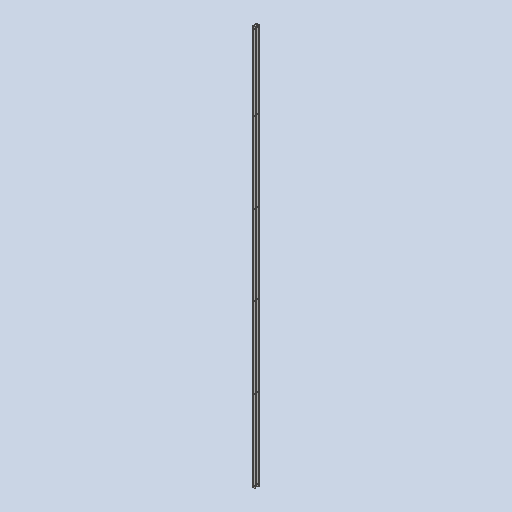
# Autodesk Inventor part: prowadnica_profil_c
Saved by Autodesk Inventor 2025.2 (Build 292293000, 293)
## iProperties
Created: 2025-03-20
Part Number: prowadnica_profil_c
Material: Ogólny
Document SubType Name: Modeling
Designer: tadek
Density: 1 g/cm^3
Appearance: Domyślna
Author: tadek
Autodesk Inventor part; units mm, degrees
ref_plane "YZ Plane" through (0, 0, 0) normal (1, 0, 0) x (0, 1, 0)
ref_plane "XZ Plane" through (0, 0, 0) normal (0, 1, 0) x (-1, 0, 0)
ref_plane "XY Plane" through (0, 0, 0) normal (0, 0, 1) x (1, 0, 0)
sketch "Szkic1" plane through (0, 0, 0) normal (0, 1, 0) x (-1, 0, 0)
  line L0 (0, 0) -> (0, -5)
  line L1 (0, -5) -> (-6, -5)
  line L2 (-6, -5) -> (-6, -3.5)
  line L3 (-6, -3.5) -> (-1.5, -3.5)
  line L4 (-1.5, -3.5) -> (-1.5, 0)
  line L5 (0, 0) -> (-1.5, 0)
  line L6 (0, 0) -> (0, 5)
  line L7 (0, 5) -> (-6, 5)
  line L8 (-6, 5) -> (-6, 3.5)
  line L9 (-6, 3.5) -> (-1.5, 3.5)
  line L10 (-1.5, 3.5) -> (-1.5, 0)
  dimension "d0" = 5
  dimension "d1" = 6
  dimension "d3" = 1.5
  dimension "d41" = 1.5
  constraints: 22 end point, 4 symmetric about line, 3 perpendicular, 2 vertical, 1 horizontal
  measures "d0" distance of L0.start L0.end
  measures "d1" distance of L0.end L1.end
  measures "d3" distance of L1.end L2.end
  measures "d41" distance between parallel lines of L0 L4
extrude "Wyciągnięcie proste1" add sketch "Szkic1" along normal blind 1000
sketch "Szkic2" plane through (1.5, 0, -3.5) normal (1, 0, 0) x (0, 0, -1)
  line L0 (-3.5, 0) -> (-3.5, 1000)
  line L1 (-7, 0) -> (-7, 1000) projected
  line L2 (-3.5, 1000) -> (-3.5, 995)
  line L3 (-3.5, 995) -> (-3.5, 795)
  line L4 (-3.5, 795) -> (-3.5, 795)
  line L5 (-3.5, 795) -> (-3.5, 695)
  line L6 (-3.5, 695) -> (-3.5, 595)
  line L7 (-3.5, 595) -> (-3.5, 495)
  line L8 (-7, 0) -> (0, 0) projected
  line L9 (-3.5, 595) -> (-3.5, 395)
  line L10 (-3.5, 395) -> (-3.5, 195)
  line L11 (-3.5, 195) -> (-3.5, 0)
  line L12 (-3.5, 0) -> (-3.5, 5)
  dimension "d7" = 5
  dimension "d13" = 200
  dimension "d14" = 200
  dimension "d16" = 200
  dimension "d17" = 200
  dimension "d18" = 195
  dimension "d19" = 5
  constraints: 20 end point, 2 vertical, 1 midpoint, 1 point on line, 11 other
  measures "d7" distance of L2.start L2.end
  measures "d13" distance of L3.end L2.end
  measures "d14" distance of L6.end L3.end
  measures "d16" distance of L6.end L9.end
  measures "d17" distance of L9.end L10.end
  measures "d18" distance of L10.end L11.end
  measures "d19" distance of L11.end L12.end
sketch "Szkic3" plane through (6, 0, 5) normal (0, 0, 1) x (1, 0, 0)
  line L0 (0, 0) -> (-6, 0) projected
  line L1 (-3, 0) -> (-3, 5)
  line L2 (-3, 5) -> (-3, 205)
  line L3 (-3, 205) -> (-3, 405)
  line L4 (-3, 405) -> (-3, 605)
  line L5 (-3, 605) -> (-3, 805)
  line L6 (-3, 805) -> (-3, 1000)
  line L7 (-3, 1000) -> (-3, 995)
  dimension "d27" = 5
  dimension "d28" = 200
  dimension "d29" = 200
  dimension "d30" = 200
  dimension "d31" = 200
  dimension "d32" = 195
  dimension "d33" = 5
  constraints: 14 end point, 6 point on line, 1 midpoint, 1 vertical
  measures "d27" distance of L1.start L1.end
  measures "d28" distance of L1.end L2.end
  measures "d29" distance of L2.end L3.end
  measures "d30" distance of L3.end L4.end
  measures "d31" distance of L4.end L5.end
  measures "d32" distance of L5.end L6.end
  measures "d33" distance of L6.end L7.end
hole "Otwór2" at (3, 5, 5) at (3, 205, 5) at (3, 405, 5) at (3, 605, 5) at (3, 805, 5) at (3, 995, 5) direction (0, 0, -1) diameter 2.5 end through all countersink diameter 3 countersink angle 90
